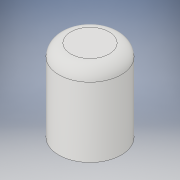
# Autodesk Inventor part: buttom piston
Saved by Autodesk Inventor 2018 (Build 220112000, 112)
## iProperties
Created: 2018-02-28
Part Number: buttom piston
Material: PBT Plastic
Document SubType Name: Modeling
Designer: 238438
Density: 1.31 g/cm^3
Appearance: Smooth - White
Mass: 0.230048 g
Surface Area: 5.91158 cm^2
Volume: 0.175609 cm^3
Author: 238438
Autodesk Inventor part; units mm, degrees
ref_plane "YZ Plane" through (0, 0, 0) normal (1, 0, 0) x (0, 1, 0)
ref_plane "XZ Plane" through (0, 0, 0) normal (0, 1, 0) x (-1, 0, 0)
ref_plane "XY Plane" through (0, 0, 0) normal (0, 0, 1) x (1, 0, 0)
sketch "Sketch1" plane through (0, 0, 0) normal (0, 1, 0) x (-1, 0, 0)
  circle A0 centre (0, 0) radius 4.1275
  dimension "d0" = 8.255
  constraints: 1 centre point, 1 coincident
  measures "d0" diameter of A0
extrude "Extrusion1" add sketch "Sketch1" along normal blind 10.795
shell "Shell1" thickness 0.635 removed faces 1 at (0.4879, 0, 1.9449)
fillet "Fillet1" radius 1.5875 1 edges at (4.1275, 10.795, 0)
body "Solid1"
